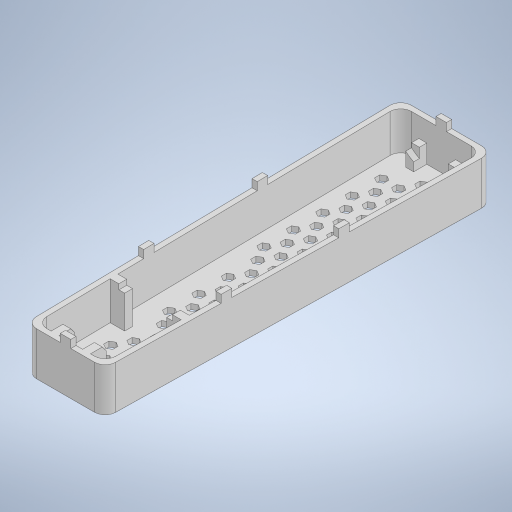
# Autodesk Inventor part: ContainerBottom
Saved by Autodesk Inventor 2023 (Build 270158000, 158)
## iProperties
Created: 2022-11-08
Part Number: ContainerBottom
Material: Generic
Document SubType Name: Modeling
Designer: The-M-Factor
Density: 1 g/cm^3
Appearance: Default
Author: The-M-Factor
Autodesk Inventor part; units mm, degrees
ref_plane "YZ Plane" through (0, 0, 0) normal (1, 0, 0) x (0, 1, 0)
ref_plane "XZ Plane" through (0, 0, 0) normal (0, 1, 0) x (-1, 0, 0)
sketch "Sketch1" plane through (0, 0, 0) normal (0, 1, 0) x (-1, 0, 0)
  line L0 (0, 0) -> (35, 0)
  line L1 (31.0843, 145) -> (2.5, 145)
  line L2 (2.5, 145) -> (32.5, 145)
  line L3 (32.5, 145) -> (35, 0)
  line L4 (0, 0) -> (2.5, 145)
  line L5 (32.9652, 2) -> (2.0348, 2)
  line L6 (2.0348, 2) -> (4.4658, 143)
  line L7 (4.4658, 143) -> (30.5342, 143)
  line L8 (30.5342, 143) -> (32.9652, 2)
  line L9 (26, 6.9925) -> (23, 6.9925)
  line L10 (26, 6.9925) -> (26, 2)
  line L11 (23, 6.9925) -> (23, 2)
  line L12 (17.5, 2) -> (17.5, 5.1674)
  line L13 (9, 6.9925) -> (12, 6.9925)
  line L14 (9, 6.9925) -> (9, 2)
  line L15 (12, 6.9925) -> (12, 2)
  line L16 (25, 137.0075) -> (22, 137.0075)
  line L17 (22, 137.0075) -> (22, 143)
  line L18 (25, 137.0075) -> (25, 143)
  line L19 (17.5, 143) -> (17.5, 140.473)
  line L20 (10, 137.0075) -> (13, 137.0075)
  line L21 (13, 137.0075) -> (13, 143)
  line L22 (10, 137.0075) -> (10, 143)
  line L23 (25.5, 114.5) -> (25.5, 111.5)
  line L24 (25.5, 111.5) -> (31.0773, 111.5)
  line L25 (25.5, 114.5) -> (31.0256, 114.5)
  line L26 (9.5, 114.5) -> (9.5, 111.5)
  line L27 (9.5, 111.5) -> (3.9227, 111.5)
  line L28 (9.5, 114.5) -> (3.9744, 114.5)
  point P0 (24.5, 6.9925)
  point P1 (23.5, 137.0075)
  point P2 (25.5, 113)
  point P3 (3.9744, 114.5)
  point P4 (3.9227, 111.5)
  point P5 (9, 2)
  point P6 (12, 2)
  dimension "d0" = 35
  dimension "d1" = 30
  dimension "d2" = 145
  dimension "d3" = 2.5
  dimension "d4" = 2
  dimension "d5" = 7
  dimension "d6" = 4.9925
  dimension "d8" = 3.1674
  dimension "d9" = 90
  dimension "d10" = 3
  dimension "d11" = 3
  dimension "d12" = 6
  dimension "d13" = 5.9925
  dimension "d14" = 3
  dimension "d15" = 30
  dimension "d16" = 8
  constraints: 58 end point, 12 symmetric about line, 7 point on line, 5 horizontal, 5 midpoint, 4 perpendicular, 2 vertical, 1 parallel, 3 other
  measures "d0" distance of L0.start L0.end
  measures "d1" distance of L1.end L2.end
  measures "d2" distance between parallel lines of L0 L1
  measures "d3" horizontal distance of L0.start L1.end
  measures "d4" distance between parallel lines of L3 L8
  measures "d5" horizontal distance of L12.start point (24.5, 6.992)
  measures "d6" vertical distance of L12.start point (24.5, 6.992)
  measures "d8" distance of L12.start L12.end
  measures "d9" angle of L5 L12
  measures "d10" distance of L16.start L16.end
  measures "d11" distance of L9.start L9.end
  measures "d12" horizontal distance of L19.start point (23.5, 137.008)
  measures "d13" vertical distance of L19.start point (23.5, 137.008)
  measures "d14" distance of L23.start L23.end
  measures "d15" vertical distance of L19.start point (25.5, 113)
  measures "d16" horizontal distance of L19.start point (25.5, 113)
extrude "Extrusion1" add sketch "Sketch1" along normal blind 2 contours L5 L10 L9 L11 L15 L13 L14 L6 L27 L26 L28 L7 L22 L20 L21 L17 L16 L18 L8 L25 L23 L24
extrude "Extrusion2" add sketch "Sketch1" along normal blind 16.5
extrude "Extrusion3" add sketch "Sketch1" along normal blind 16.5 contours L24 L23 L25 L8
extrude "Extrusion4" add sketch "Sketch1" along normal blind 16.5 contours L6 L28 L26 L27
extrude "Extrusion5" add sketch "Sketch1" along normal blind 16.5 contours L18 L16 L17 L7
extrude "Extrusion6" add sketch "Sketch1" along normal blind 16.5 contours L21 L20 L22 L7
extrude "Extrusion7" add sketch "Sketch1" along normal blind 9 contours L5 L11 L9 L10
extrude "Extrusion8" add sketch "Sketch1" along normal blind 9 contours L5 L14 L13 L15
sketch "Sketch2" plane through (0, 16.5, 0) normal (0, 1, 0) x (1, 0, 0)
  line L0 (-31.0256, -114.5) -> (-25.5, -114.5) projected
  line L1 (-27.7, -114.5) -> (-27.7, -111.5)
  line L2 (-25.5, -111.5) -> (-31.0773, -111.5) projected
  line L3 (-25.5, -114.5) -> (-25.5, -111.5) projected
  line L4 (-9.5, -114.5) -> (-3.9744, -114.5) projected
  line L5 (-7.3, -114.5) -> (-7.3, -111.5)
  line L6 (-3.9227, -111.5) -> (-9.5, -111.5) projected
  line L7 (-9.5, -111.5) -> (-9.5, -114.5) projected
  point P0 (0, 0)
  dimension "d33" = 2.2
  dimension "d34" = 2.2
  constraints: 4 end point, 4 point on line, 2 vertical
  measures "d33" distance between parallel lines of L3 L1
  measures "d34" distance between parallel lines of L7 L5
extrude "Extrusion9" cut sketch "Sketch2" against normal blind 2 contours L1 L2 L3 L0
extrude "Extrusion10" cut sketch "Sketch2" against normal blind 2 contours L7 L6 L5 L4
chamfer "Chamfer1" distance 1.5 distance2 2 1 edges at (-11.5, 16.5, 137.0075) measured on face at (-2.1409, 16.5, 85.5)
chamfer "Chamfer2" distance 1.5 distance2 2 1 edges at (-23.5, 16.5, 137.0075) measured on face at (-2.1409, 16.5, 85.5)
ref_plane "Work Plane1" through (0, 0, 6.9925) normal (0, 0, 1) x (1, 0, 0)
sketch "Sketch3" plane through (0, 0, 6.9925) normal (0, 0, 1) x (1, 0, 0)
  line L0 (-12, 2) -> (-12, 9) projected
  line L1 (-23, 2) -> (-12, 2)
  line L2 (-17.5, 2) -> (-17.5, 16.5)
  circle A0 centre (-17.5, 16.5) radius 12.5
  point P0 (0, 0)
  dimension "d46" = 14.5
  dimension "d47" = 25
  constraints: 4 end point, 1 centre point, 1 coincident, 1 horizontal, 1 midpoint, 1 vertical
  measures "d46" distance of L2.start L2.end
  measures "d47" diameter of A0
extrude "Extrusion11" cut sketch "Sketch3" against normal blind 2.2 contours A0
sketch "Sketch5" plane through (0, 2, 0) normal (0, 1, 0) x (1, 0, 0)
  line L0 (-17, -131) -> (-15.2679, -132)
  line L1 (-15.2679, -132) -> (-15.2679, -134)
  line L2 (-15.2679, -134) -> (-17, -135)
  line L3 (-17, -135) -> (-18.7321, -134)
  line L4 (-18.7321, -134) -> (-18.7321, -132)
  line L5 (-18.7321, -132) -> (-17, -131)
  line L6 (-22, -137.0075) -> (-22, -143) projected
  line L7 (-22, -143) -> (-13, -143) projected
  line L8 (-22.1856, -132.2619) -> (-19.9814, -130.9893)
  line L9 (-14.5757, -130.6676) -> (-12.1577, -132.0636)
  line L10 (-18.7321, -133) -> (-19.3956, -133)
  line L11 (-25.5, -111.5) -> (-25.5, -114.5) projected
  line L12 (-32.9652, -2) -> (-31.0773, -111.5) projected
  line L13 (-15.5, -128.4019) -> (-13.7679, -129.4019)
  line L14 (-13.7679, -129.4019) -> (-12.0359, -128.4019)
  line L15 (-12.0359, -128.4019) -> (-12.0359, -126.4019)
  line L16 (-12.0359, -126.4019) -> (-13.7679, -125.4019)
  line L17 (-13.7679, -125.4019) -> (-15.5, -126.4019)
  line L18 (-15.5, -126.4019) -> (-15.5, -128.4019)
  line L19 (-18.5, -128.4019) -> (-18.5, -126.4019)
  line L20 (-18.5, -126.4019) -> (-20.2321, -125.4019)
  line L21 (-20.2321, -125.4019) -> (-21.9641, -126.4019)
  line L22 (-21.9641, -126.4019) -> (-21.9641, -128.4019)
  line L23 (-21.9641, -128.4019) -> (-20.2321, -129.4019)
  line L24 (-20.2321, -129.4019) -> (-18.5, -128.4019)
  line L25 (-18.2258, -127.4019) -> (-16.8285, -127.4019)
  line L26 (-17, -123.8038) -> (-15.2679, -122.8038)
  line L27 (-15.2679, -122.8038) -> (-15.2679, -120.8038)
  line L28 (-15.2679, -120.8038) -> (-17, -119.8038)
  line L29 (-17, -119.8038) -> (-18.7321, -120.8038)
  line L30 (-18.7321, -120.8038) -> (-18.7321, -122.8038)
  line L31 (-18.7321, -122.8038) -> (-17, -123.8038)
  line L32 (-18.7321, -121.8038) -> (-20.5, -121.8038)
  line L33 (-17, -112.6077) -> (-15.2679, -111.6077)
  line L34 (-15.2679, -111.6077) -> (-15.2679, -109.6077)
  line L35 (-15.2679, -109.6077) -> (-17, -108.6077)
  line L36 (-17, -108.6077) -> (-18.7321, -109.6077)
  line L37 (-18.7321, -109.6077) -> (-18.7321, -111.6077)
  line L38 (-18.7321, -111.6077) -> (-17, -112.6077)
  line L39 (-22.1856, -111.3458) -> (-19.9814, -112.6184)
  line L40 (-14.5757, -112.9401) -> (-12.1577, -111.5441)
  line L41 (-18.7321, -110.6077) -> (-19.3956, -110.6077)
  line L42 (-13.7679, -118.2058) -> (-15.5, -117.2058)
  line L43 (-12.0359, -117.2058) -> (-13.7679, -118.2058)
  line L44 (-12.0359, -115.2058) -> (-12.0359, -117.2058)
  line L45 (-13.7679, -114.2058) -> (-12.0359, -115.2058)
  line L46 (-15.5, -115.2058) -> (-13.7679, -114.2058)
  line L47 (-15.5, -117.2058) -> (-15.5, -115.2058)
  line L48 (-21.9641, -115.2058) -> (-20.2321, -114.2058)
  line L49 (-21.9641, -117.2058) -> (-21.9641, -115.2058)
  line L50 (-20.2321, -118.2058) -> (-21.9641, -117.2058)
  line L51 (-18.5, -117.2058) -> (-20.2321, -118.2058)
  line L52 (-18.5, -115.2058) -> (-18.5, -117.2058)
  line L53 (-20.2321, -114.2058) -> (-18.5, -115.2058)
  line L54 (-18.2258, -116.2058) -> (-16.8285, -116.2058)
  line L55 (-18.7321, -98.4115) -> (-17, -97.4115)
  line L56 (-18.7321, -100.4115) -> (-18.7321, -98.4115)
  line L57 (-17, -101.4115) -> (-18.7321, -100.4115)
  line L58 (-15.2679, -100.4115) -> (-17, -101.4115)
  line L59 (-15.2679, -98.4115) -> (-15.2679, -100.4115)
  line L60 (-17, -97.4115) -> (-15.2679, -98.4115)
  line L61 (-18.7321, -99.4115) -> (-20.5, -99.4115)
  line L62 (-21.9641, -104.0096) -> (-21.9641, -106.0096)
  line L63 (-18.5, -104.0096) -> (-20.2321, -103.0096)
  line L64 (-20.2321, -103.0096) -> (-21.9641, -104.0096)
  line L65 (-21.9641, -106.0096) -> (-20.2321, -107.0096)
  line L66 (-18.5, -106.0096) -> (-18.5, -104.0096)
  line L67 (-20.2321, -107.0096) -> (-18.5, -106.0096)
  line L68 (-18.2258, -105.0096) -> (-16.8285, -105.0096)
  line L69 (-13.7679, -107.0096) -> (-12.0359, -106.0096)
  line L70 (-13.7679, -103.0096) -> (-15.5, -104.0096)
  line L71 (-12.0359, -106.0096) -> (-12.0359, -104.0096)
  line L72 (-12.0359, -104.0096) -> (-13.7679, -103.0096)
  line L73 (-15.5, -106.0096) -> (-13.7679, -107.0096)
  line L74 (-15.5, -104.0096) -> (-15.5, -106.0096)
  line L75 (-22.1856, -109.8696) -> (-19.9814, -108.597)
  line L76 (-14.5757, -108.2753) -> (-12.1577, -109.6713)
  line L77 (-18.7321, -76.0192) -> (-17, -75.0192)
  line L78 (-18.7321, -78.0192) -> (-18.7321, -76.0192)
  line L79 (-17, -79.0192) -> (-18.7321, -78.0192)
  line L80 (-15.2679, -78.0192) -> (-17, -79.0192)
  line L81 (-15.2679, -76.0192) -> (-15.2679, -78.0192)
  line L82 (-17, -75.0192) -> (-15.2679, -76.0192)
  line L83 (-18.7321, -77.0192) -> (-20.5, -77.0192)
  line L84 (-21.9641, -81.6173) -> (-21.9641, -83.6173)
  line L85 (-18.5, -81.6173) -> (-20.2321, -80.6173)
  line L86 (-20.2321, -80.6173) -> (-21.9641, -81.6173)
  line L87 (-21.9641, -83.6173) -> (-20.2321, -84.6173)
  line L88 (-18.5, -83.6173) -> (-18.5, -81.6173)
  line L89 (-20.2321, -84.6173) -> (-18.5, -83.6173)
  line L90 (-18.2258, -82.6173) -> (-16.8285, -82.6173)
  line L91 (-13.7679, -84.6173) -> (-12.0359, -83.6173)
  line L92 (-13.7679, -80.6173) -> (-15.5, -81.6173)
  line L93 (-12.0359, -83.6173) -> (-12.0359, -81.6173)
  line L94 (-12.0359, -81.6173) -> (-13.7679, -80.6173)
  line L95 (-15.5, -83.6173) -> (-13.7679, -84.6173)
  line L96 (-15.5, -81.6173) -> (-15.5, -83.6173)
  line L97 (-22.1856, -87.4773) -> (-19.9814, -86.2047)
  line L98 (-14.5757, -85.883) -> (-12.1577, -87.279)
  line L99 (-17, -86.2154) -> (-15.2679, -87.2154)
  line L100 (-18.7321, -87.2154) -> (-17, -86.2154)
  line L101 (-18.7321, -89.2154) -> (-18.7321, -87.2154)
  line L102 (-17, -90.2154) -> (-18.7321, -89.2154)
  line L103 (-15.2679, -89.2154) -> (-17, -90.2154)
  line L104 (-15.2679, -87.2154) -> (-15.2679, -89.2154)
  line L105 (-18.7321, -88.2154) -> (-19.3956, -88.2154)
  line L106 (-20.2321, -95.8135) -> (-21.9641, -94.8135)
  line L107 (-18.5, -94.8135) -> (-20.2321, -95.8135)
  line L108 (-14.5757, -90.5478) -> (-12.1577, -89.1518)
  line L109 (-15.5, -92.8135) -> (-13.7679, -91.8135)
  line L110 (-13.7679, -95.8135) -> (-15.5, -94.8135)
  line L111 (-12.0359, -94.8135) -> (-13.7679, -95.8135)
  line L112 (-12.0359, -92.8135) -> (-12.0359, -94.8135)
  line L113 (-13.7679, -91.8135) -> (-12.0359, -92.8135)
  line L114 (-15.5, -94.8135) -> (-15.5, -92.8135)
  line L115 (-18.2258, -93.8135) -> (-16.8285, -93.8135)
  line L116 (-21.9641, -94.8135) -> (-21.9641, -92.8135)
  line L117 (-18.5, -92.8135) -> (-18.5, -94.8135)
  line L118 (-21.9641, -92.8135) -> (-20.2321, -91.8135)
  line L119 (-20.2321, -91.8135) -> (-18.5, -92.8135)
  line L120 (-22.1856, -88.9535) -> (-19.9814, -90.2261)
  line L121 (-18.7321, -31.2346) -> (-17, -30.2346)
  line L122 (-18.7321, -33.2346) -> (-18.7321, -31.2346)
  line L123 (-17, -34.2346) -> (-18.7321, -33.2346)
  line L124 (-15.2679, -33.2346) -> (-17, -34.2346)
  line L125 (-15.2679, -31.2346) -> (-15.2679, -33.2346)
  line L126 (-17, -30.2346) -> (-15.2679, -31.2346)
  line L127 (-18.7321, -32.2346) -> (-20.5, -32.2346)
  line L128 (-21.9641, -36.8327) -> (-21.9641, -38.8327)
  line L129 (-18.5, -36.8327) -> (-20.2321, -35.8327)
  line L130 (-20.2321, -35.8327) -> (-21.9641, -36.8327)
  line L131 (-21.9641, -38.8327) -> (-20.2321, -39.8327)
  line L132 (-18.5, -38.8327) -> (-18.5, -36.8327)
  line L133 (-20.2321, -39.8327) -> (-18.5, -38.8327)
  line L134 (-18.2258, -37.8327) -> (-16.8285, -37.8327)
  line L135 (-13.7679, -39.8327) -> (-12.0359, -38.8327)
  line L136 (-13.7679, -35.8327) -> (-15.5, -36.8327)
  line L137 (-12.0359, -38.8327) -> (-12.0359, -36.8327)
  line L138 (-12.0359, -36.8327) -> (-13.7679, -35.8327)
  line L139 (-15.5, -38.8327) -> (-13.7679, -39.8327)
  line L140 (-15.5, -36.8327) -> (-15.5, -38.8327)
  line L141 (-22.1856, -42.6927) -> (-19.9814, -41.4201)
  line L142 (-14.5757, -41.0984) -> (-12.1577, -42.4944)
  line L143 (-17, -41.4308) -> (-15.2679, -42.4308)
  line L144 (-18.7321, -42.4308) -> (-17, -41.4308)
  line L145 (-18.7321, -44.4308) -> (-18.7321, -42.4308)
  line L146 (-17, -45.4308) -> (-18.7321, -44.4308)
  line L147 (-15.2679, -44.4308) -> (-17, -45.4308)
  line L148 (-15.2679, -42.4308) -> (-15.2679, -44.4308)
  line L149 (-18.7321, -43.4308) -> (-19.3956, -43.4308)
  line L150 (-18.7321, -55.6269) -> (-17, -56.6269)
  line L151 (-17, -56.6269) -> (-15.2679, -55.6269)
  line L152 (-18.7321, -54.6269) -> (-20.5, -54.6269)
  line L153 (-18.7321, -53.6269) -> (-18.7321, -55.6269)
  line L154 (-15.2679, -55.6269) -> (-15.2679, -53.6269)
  line L155 (-15.2679, -53.6269) -> (-17, -52.6269)
  line L156 (-17, -52.6269) -> (-18.7321, -53.6269)
  line L157 (-20.2321, -51.0289) -> (-21.9641, -50.0289)
  line L158 (-18.5, -50.0289) -> (-20.2321, -51.0289)
  line L159 (-14.5757, -45.7632) -> (-12.1577, -44.3671)
  line L160 (-15.5, -48.0289) -> (-13.7679, -47.0289)
  line L161 (-13.7679, -51.0289) -> (-15.5, -50.0289)
  line L162 (-12.0359, -50.0289) -> (-13.7679, -51.0289)
  line L163 (-12.0359, -48.0289) -> (-12.0359, -50.0289)
  line L164 (-13.7679, -47.0289) -> (-12.0359, -48.0289)
  line L165 (-15.5, -50.0289) -> (-15.5, -48.0289)
  line L166 (-18.2258, -49.0289) -> (-16.8285, -49.0289)
  line L167 (-21.9641, -50.0289) -> (-21.9641, -48.0289)
  line L168 (-18.5, -48.0289) -> (-18.5, -50.0289)
  line L169 (-21.9641, -48.0289) -> (-20.2321, -47.0289)
  line L170 (-20.2321, -47.0289) -> (-18.5, -48.0289)
  line L171 (-22.1856, -44.1689) -> (-19.9814, -45.4415)
  line L172 (-20.2321, -69.4212) -> (-18.5, -70.4212)
  line L173 (-21.9641, -70.4212) -> (-20.2321, -69.4212)
  line L174 (-18.5, -72.4212) -> (-20.2321, -73.4212)
  line L175 (-21.9641, -72.4212) -> (-21.9641, -70.4212)
  line L176 (-20.2321, -73.4212) -> (-21.9641, -72.4212)
  line L177 (-18.5, -61.225) -> (-18.5, -59.225)
  line L178 (-22.1856, -65.085) -> (-19.9814, -63.8124)
  line L179 (-18.2258, -71.4212) -> (-16.8285, -71.4212)
  line L180 (-18.5, -70.4212) -> (-18.5, -72.4212)
  line L181 (-13.7679, -73.4212) -> (-15.5, -72.4212)
  line L182 (-12.0359, -72.4212) -> (-13.7679, -73.4212)
  line L183 (-15.5, -72.4212) -> (-15.5, -70.4212)
  line L184 (-12.0359, -70.4212) -> (-12.0359, -72.4212)
  line L185 (-15.5, -70.4212) -> (-13.7679, -69.4212)
  line L186 (-13.7679, -69.4212) -> (-12.0359, -70.4212)
  line L187 (-22.1856, -66.5612) -> (-19.9814, -67.8338)
  line L188 (-18.7321, -66.8231) -> (-17, -67.8231)
  line L189 (-14.5757, -68.1555) -> (-12.1577, -66.7594)
  line L190 (-17, -67.8231) -> (-15.2679, -66.8231)
  line L191 (-18.7321, -64.8231) -> (-18.7321, -66.8231)
  line L192 (-15.2679, -66.8231) -> (-15.2679, -64.8231)
  line L193 (-17, -63.8231) -> (-18.7321, -64.8231)
  line L194 (-15.2679, -64.8231) -> (-17, -63.8231)
  line L195 (-18.7321, -65.8231) -> (-19.3956, -65.8231)
  line L196 (-18.5, -59.225) -> (-20.2321, -58.225)
  line L197 (-20.2321, -58.225) -> (-21.9641, -59.225)
  line L198 (-21.9641, -61.225) -> (-20.2321, -62.225)
  line L199 (-21.9641, -59.225) -> (-21.9641, -61.225)
  line L200 (-20.2321, -62.225) -> (-18.5, -61.225)
  line L201 (-14.5757, -63.4907) -> (-12.1577, -64.8867)
  line L202 (-18.2258, -60.225) -> (-16.8285, -60.225)
  line L203 (-15.5, -61.225) -> (-13.7679, -62.225)
  line L204 (-13.7679, -62.225) -> (-12.0359, -61.225)
  line L205 (-15.5, -59.225) -> (-15.5, -61.225)
  line L206 (-12.0359, -61.225) -> (-12.0359, -59.225)
  line L207 (-12.0359, -59.225) -> (-13.7679, -58.225)
  line L208 (-13.7679, -58.225) -> (-15.5, -59.225)
  line L209 (-18.5, -27.6366) -> (-20.2321, -28.6366)
  line L210 (-20.2321, -28.6366) -> (-21.9641, -27.6366)
  line L211 (-21.9641, -27.6366) -> (-21.9641, -25.6366)
  line L212 (-20.2321, -24.6366) -> (-18.5, -25.6366)
  line L213 (-21.9641, -25.6366) -> (-20.2321, -24.6366)
  line L214 (-22.1856, -21.7766) -> (-19.9814, -23.0492)
  line L215 (-18.7321, -22.0385) -> (-17, -23.0385)
  line L216 (-18.7321, -21.0385) -> (-19.3956, -21.0385)
  line L217 (-14.5757, -23.3709) -> (-12.1577, -21.9748)
  line L218 (-18.7321, -20.0385) -> (-18.7321, -22.0385)
  line L219 (-17, -23.0385) -> (-15.2679, -22.0385)
  line L220 (-15.2679, -22.0385) -> (-15.2679, -20.0385)
  line L221 (-17, -19.0385) -> (-18.7321, -20.0385)
  line L222 (-15.2679, -20.0385) -> (-17, -19.0385)
  line L223 (-22.1856, -20.3004) -> (-19.9814, -19.0278)
  line L224 (-18.2258, -15.4404) -> (-16.8285, -15.4404)
  line L225 (-20.2321, -17.4404) -> (-18.5, -16.4404)
  line L226 (-21.9641, -16.4404) -> (-20.2321, -17.4404)
  line L227 (-18.5, -16.4404) -> (-18.5, -14.4404)
  line L228 (-18.5, -14.4404) -> (-20.2321, -13.4404)
  line L229 (-21.9641, -14.4404) -> (-21.9641, -16.4404)
  line L230 (-20.2321, -13.4404) -> (-21.9641, -14.4404)
  line L231 (-18.5, -25.6366) -> (-18.5, -27.6366)
  line L232 (-18.2258, -26.6366) -> (-16.8285, -26.6366)
  line L233 (-15.5, -25.6366) -> (-13.7679, -24.6366)
  line L234 (-15.5, -27.6366) -> (-15.5, -25.6366)
  line L235 (-13.7679, -28.6366) -> (-15.5, -27.6366)
  line L236 (-12.0359, -25.6366) -> (-12.0359, -27.6366)
  line L237 (-12.0359, -27.6366) -> (-13.7679, -28.6366)
  line L238 (-13.7679, -24.6366) -> (-12.0359, -25.6366)
  line L239 (-18.7321, -8.8423) -> (-17, -7.8423)
  line L240 (-17, -7.8423) -> (-15.2679, -8.8423)
  line L241 (-18.7321, -9.8423) -> (-20.5, -9.8423)
  line L242 (-18.7321, -10.8423) -> (-18.7321, -8.8423)
  line L243 (-15.2679, -8.8423) -> (-15.2679, -10.8423)
  line L244 (-15.2679, -10.8423) -> (-17, -11.8423)
  line L245 (-17, -11.8423) -> (-18.7321, -10.8423)
  line L246 (-14.5757, -18.7061) -> (-12.1577, -20.1021)
  line L247 (-15.5, -16.4404) -> (-13.7679, -17.4404)
  line L248 (-15.5, -14.4404) -> (-15.5, -16.4404)
  line L249 (-13.7679, -17.4404) -> (-12.0359, -16.4404)
  line L250 (-12.0359, -16.4404) -> (-12.0359, -14.4404)
  line L251 (-12.0359, -14.4404) -> (-13.7679, -13.4404)
  line L252 (-13.7679, -13.4404) -> (-15.5, -14.4404)
  line L253 (-25.5, -114.5) -> (-31.0256, -114.5) projected
  point P0 (0, 0)
  point P1 (-17, -133)
  point P2 (-21.0835, -131.6256)
  point P3 (-19.0638, -133)
  dimension "d55" = 2
  dimension "d59" = 1.5
  dimension "d60" = 1.5
  dimension "d63" = 2.0638
  dimension "d170" = 3.5981
  dimension "d184" = 8.5
  dimension "d185" = 18.5
  dimension "d186" = 90
  constraints: 498 end point, 278 symmetric about line, 4 midpoint, 3 horizontal, 2 parallel, 13 other
  measures "d55" distance of L0.end L1.end
  measures "d59" distance from line of L5 point (-21.084, -131.626)
  measures "d60" distance between parallel lines of L0 L9
  measures "d63" horizontal distance of L0.start point (-19.064, -133)
  measures "d170" vertical distance of L0.start L25.start
  measures "d184" distance from line of L11 point (-17, -133)
  measures "d185" distance from line of L253 point (-17, -133)
  measures "d186" angle of L253 L4
fillet "Fillet1" radius 4 2 edges at (-35, 8.25, 0) (0, 8.25, 0)
fillet "Fillet2" radius 4 1 edges at (-32.9652, 9.25, 2)
fillet "Fillet3" radius 4 1 edges at (-2.0348, 9.25, 2)
fillet "Fillet4" radius 4 2 edges at (-32.5, 8.25, 145) (-2.5, 8.25, 145)
fillet "Fillet5" radius 4 1 edges at (-30.5342, 9.25, 143)
fillet "Fillet6" radius 4 1 edges at (-4.4658, 9.25, 143)
extrude "CenterHoles" cut sketch "Sketch5" against normal blind 2
sketch "Sketch8" plane through (0, 2, 0) normal (0, 1, 0) x (1, 0, 0)
  line L0 (-24.9641, -14.4404) -> (-24.9641, -16.4404)
  line L1 (-24.9641, -16.4404) -> (-26.6962, -17.4404)
  line L2 (-26.6962, -17.4404) -> (-28.4282, -16.4404)
  line L3 (-28.4282, -16.4404) -> (-28.4282, -14.4404)
  line L4 (-28.4282, -14.4404) -> (-26.6962, -13.4404)
  line L5 (-26.6962, -13.4404) -> (-24.9641, -14.4404)
  line L6 (-26, -6.9925) -> (-26, -4.7925) projected
  line L7 (-21.9641, -16.4404) -> (-21.9641, -14.4404) projected
  line L8 (-26.8244, -19.2465) -> (-24.0082, -17.6206)
  line L9 (-21.7321, -20.0385) -> (-23.4641, -19.0385)
  line L10 (-23.4641, -19.0385) -> (-25.1962, -20.0385)
  line L11 (-25.1962, -20.0385) -> (-25.1962, -22.0385)
  line L12 (-25.1962, -22.0385) -> (-23.4641, -23.0385)
  line L13 (-23.4641, -23.0385) -> (-21.7321, -22.0385)
  line L14 (-21.7321, -22.0385) -> (-21.7321, -20.0385)
  line L15 (-25.1962, -21.0385) -> (-26.7131, -21.0385)
  line L16 (-24.9641, -27.6366) -> (-24.9641, -25.6366)
  line L17 (-24.9641, -25.6366) -> (-26.6962, -24.6366)
  line L18 (-26.6962, -24.6366) -> (-28.4282, -25.6366)
  line L19 (-28.4282, -25.6366) -> (-28.4282, -27.6366)
  line L20 (-28.4282, -27.6366) -> (-26.6962, -28.6366)
  line L21 (-26.6962, -28.6366) -> (-24.9641, -27.6366)
  line L22 (-26.8244, -22.8304) -> (-24.0082, -24.4564)
  line L23 (-24.9641, -26.6366) -> (-24.1308, -26.6366)
  line L24 (-24.9641, -38.8327) -> (-24.9641, -36.8327)
  line L25 (-24.9641, -36.8327) -> (-26.6962, -35.8327)
  line L26 (-26.6962, -35.8327) -> (-28.4282, -36.8327)
  line L27 (-28.4282, -36.8327) -> (-28.4282, -38.8327)
  line L28 (-28.4282, -38.8327) -> (-26.6962, -39.8327)
  line L29 (-26.6962, -39.8327) -> (-24.9641, -38.8327)
  line L30 (-26.8244, -34.0266) -> (-24.0082, -35.6525)
  line L31 (-21.7321, -31.2346) -> (-21.7321, -33.2346)
  line L32 (-21.7321, -33.2346) -> (-23.4641, -34.2346)
  line L33 (-23.4641, -34.2346) -> (-25.1962, -33.2346)
  line L34 (-25.1962, -33.2346) -> (-25.1962, -31.2346)
  line L35 (-25.1962, -31.2346) -> (-23.4641, -30.2346)
  line L36 (-23.4641, -30.2346) -> (-21.7321, -31.2346)
  line L37 (-25.1962, -32.2346) -> (-26.7131, -32.2346)
  line L38 (-26.8244, -30.4427) -> (-24.0082, -28.8167)
  line L39 (-24.9641, -37.8327) -> (-24.1308, -37.8327)
  line L40 (-21.7321, -53.6269) -> (-21.7321, -55.6269)
  line L41 (-21.7321, -55.6269) -> (-23.4641, -56.6269)
  line L42 (-23.4641, -56.6269) -> (-25.1962, -55.6269)
  line L43 (-25.1962, -55.6269) -> (-25.1962, -53.6269)
  line L44 (-25.1962, -53.6269) -> (-23.4641, -52.6269)
  line L45 (-23.4641, -52.6269) -> (-21.7321, -53.6269)
  line L46 (-25.1962, -54.6269) -> (-26.7131, -54.6269)
  line L47 (-28.4282, -50.0289) -> (-28.4282, -48.0289)
  line L48 (-28.4282, -48.0289) -> (-26.6962, -47.0289)
  line L49 (-26.6962, -47.0289) -> (-24.9641, -48.0289)
  line L50 (-24.9641, -48.0289) -> (-24.9641, -50.0289)
  line L51 (-24.9641, -50.0289) -> (-26.6962, -51.0289)
  line L52 (-26.6962, -51.0289) -> (-28.4282, -50.0289)
  line L53 (-26.8244, -52.835) -> (-24.0082, -51.209)
  line L54 (-24.9641, -49.0289) -> (-24.1308, -49.0289)
  line L55 (-26.8244, -41.6388) -> (-24.0082, -40.0129)
  line L56 (-25.1962, -43.4308) -> (-26.7131, -43.4308)
  line L57 (-26.8244, -45.2228) -> (-24.0082, -46.8487)
  line L58 (-25.1962, -44.4308) -> (-23.4641, -45.4308)
  line L59 (-25.1962, -42.4308) -> (-25.1962, -44.4308)
  line L60 (-23.4641, -41.4308) -> (-25.1962, -42.4308)
  line L61 (-21.7321, -42.4308) -> (-23.4641, -41.4308)
  line L62 (-21.7321, -44.4308) -> (-21.7321, -42.4308)
  line L63 (-23.4641, -45.4308) -> (-21.7321, -44.4308)
  line L64 (-26.8244, -56.4189) -> (-24.0082, -58.0448)
  line L65 (-24.9641, -60.225) -> (-24.1308, -60.225)
  line L66 (-28.4282, -61.225) -> (-26.6962, -62.225)
  line L67 (-26.6962, -62.225) -> (-24.9641, -61.225)
  line L68 (-24.9641, -61.225) -> (-24.9641, -59.225)
  line L69 (-26.6962, -58.225) -> (-28.4282, -59.225)
  line L70 (-24.9641, -59.225) -> (-26.6962, -58.225)
  line L71 (-28.4282, -59.225) -> (-28.4282, -61.225)
  line L72 (-25.1962, -64.8231) -> (-23.4641, -63.8231)
  line L73 (-23.4641, -63.8231) -> (-21.7321, -64.8231)
  line L74 (-25.1962, -65.8231) -> (-26.7131, -65.8231)
  line L75 (-25.1962, -66.8231) -> (-25.1962, -64.8231)
  line L76 (-21.7321, -64.8231) -> (-21.7321, -66.8231)
  line L77 (-21.7321, -66.8231) -> (-23.4641, -67.8231)
  line L78 (-23.4641, -67.8231) -> (-25.1962, -66.8231)
  line L79 (-23.4641, -75.0192) -> (-25.1962, -76.0192)
  line L80 (-21.7321, -76.0192) -> (-23.4641, -75.0192)
  line L81 (-25.1962, -77.0192) -> (-26.7131, -77.0192)
  line L82 (-21.7321, -78.0192) -> (-21.7321, -76.0192)
  line L83 (-23.4641, -79.0192) -> (-21.7321, -78.0192)
  line L84 (-25.1962, -76.0192) -> (-25.1962, -78.0192)
  line L85 (-25.1962, -78.0192) -> (-23.4641, -79.0192)
  line L86 (-25.1962, -87.2154) -> (-23.4641, -86.2154)
  line L87 (-23.4641, -86.2154) -> (-21.7321, -87.2154)
  line L88 (-25.1962, -88.2154) -> (-26.7131, -88.2154)
  line L89 (-25.1962, -89.2154) -> (-25.1962, -87.2154)
  line L90 (-21.7321, -87.2154) -> (-21.7321, -89.2154)
  line L91 (-21.7321, -89.2154) -> (-23.4641, -90.2154)
  line L92 (-23.4641, -90.2154) -> (-25.1962, -89.2154)
  line L93 (-23.4641, -101.4115) -> (-25.1962, -100.4115)
  line L94 (-25.1962, -98.4115) -> (-23.4641, -97.4115)
  line L95 (-25.1962, -99.4115) -> (-26.7131, -99.4115)
  line L96 (-23.4641, -97.4115) -> (-21.7321, -98.4115)
  line L97 (-25.1962, -100.4115) -> (-25.1962, -98.4115)
  line L98 (-21.7321, -100.4115) -> (-23.4641, -101.4115)
  line L99 (-21.7321, -98.4115) -> (-21.7321, -100.4115)
  line L100 (-17, -75.0192) -> (-17, -73.4581)
  line L101 (-15.2679, -76.0192) -> (-15.2679, -78.0192) projected
  line L102 (-23.4641, -123.8038) -> (-25.1962, -122.8038)
  line L103 (-25.1962, -120.8038) -> (-23.4641, -119.8038)
  line L104 (-25.1962, -121.8038) -> (-26.7131, -121.8038)
  line L105 (-23.4641, -119.8038) -> (-21.7321, -120.8038)
  line L106 (-25.1962, -122.8038) -> (-25.1962, -120.8038)
  line L107 (-21.7321, -122.8038) -> (-23.4641, -123.8038)
  line L108 (-21.7321, -120.8038) -> (-21.7321, -122.8038)
  line L109 (-9.0359, -14.4404) -> (-9.0359, -16.4404)
  line L110 (-9.0359, -16.4404) -> (-7.3038, -17.4404)
  line L111 (-7.3038, -17.4404) -> (-5.5718, -16.4404)
  line L112 (-5.5718, -16.4404) -> (-5.5718, -14.4404)
  line L113 (-5.5718, -14.4404) -> (-7.3038, -13.4404)
  line L114 (-7.3038, -13.4404) -> (-9.0359, -14.4404)
  line L115 (-7.1756, -19.2465) -> (-9.9918, -17.6206)
  line L116 (-12.2679, -22.0385) -> (-12.2679, -20.0385)
  line L117 (-12.2679, -20.0385) -> (-10.5359, -19.0385)
  line L118 (-10.5359, -19.0385) -> (-8.8038, -20.0385)
  line L119 (-8.8038, -20.0385) -> (-8.8038, -22.0385)
  line L120 (-8.8038, -22.0385) -> (-10.5359, -23.0385)
  line L121 (-10.5359, -23.0385) -> (-12.2679, -22.0385)
  line L122 (-8.8038, -21.0385) -> (-7.2869, -21.0385)
  line L123 (-5.5718, -25.6366) -> (-5.5718, -27.6366)
  line L124 (-5.5718, -27.6366) -> (-7.3038, -28.6366)
  line L125 (-7.3038, -28.6366) -> (-9.0359, -27.6366)
  line L126 (-9.0359, -27.6366) -> (-9.0359, -25.6366)
  line L127 (-9.0359, -25.6366) -> (-7.3038, -24.6366)
  line L128 (-7.3038, -24.6366) -> (-5.5718, -25.6366)
  line L129 (-7.1756, -22.8304) -> (-9.9918, -24.4564)
  line L130 (-9.0359, -26.6366) -> (-9.8692, -26.6366)
  line L131 (-9.0359, -38.8327) -> (-9.0359, -36.8327)
  line L132 (-7.3038, -39.8327) -> (-9.0359, -38.8327)
  line L133 (-5.5718, -38.8327) -> (-7.3038, -39.8327)
  line L134 (-5.5718, -36.8327) -> (-5.5718, -38.8327)
  line L135 (-7.3038, -35.8327) -> (-5.5718, -36.8327)
  line L136 (-9.0359, -36.8327) -> (-7.3038, -35.8327)
  line L137 (-7.1756, -34.0266) -> (-9.9918, -35.6525)
  line L138 (-8.8038, -32.2346) -> (-7.2869, -32.2346)
  line L139 (-7.1756, -30.4427) -> (-9.9918, -28.8167)
  line L140 (-8.8038, -31.2346) -> (-10.5359, -30.2346)
  line L141 (-8.8038, -33.2346) -> (-8.8038, -31.2346)
  line L142 (-10.5359, -34.2346) -> (-8.8038, -33.2346)
  line L143 (-12.2679, -33.2346) -> (-10.5359, -34.2346)
  line L144 (-12.2679, -31.2346) -> (-12.2679, -33.2346)
  line L145 (-10.5359, -30.2346) -> (-12.2679, -31.2346)
  line L146 (-9.0359, -37.8327) -> (-9.8692, -37.8327)
  line L147 (-10.5359, -56.6269) -> (-8.8038, -55.6269)
  line L148 (-12.2679, -55.6269) -> (-10.5359, -56.6269)
  line L149 (-8.8038, -54.6269) -> (-7.2869, -54.6269)
  line L150 (-12.2679, -53.6269) -> (-12.2679, -55.6269)
  line L151 (-10.5359, -52.6269) -> (-12.2679, -53.6269)
  line L152 (-8.8038, -55.6269) -> (-8.8038, -53.6269)
  line L153 (-8.8038, -53.6269) -> (-10.5359, -52.6269)
  line L154 (-7.1756, -52.835) -> (-9.9918, -51.209)
  line L155 (-9.0359, -49.0289) -> (-9.8692, -49.0289)
  line L156 (-5.5718, -48.0289) -> (-7.3038, -47.0289)
  line L157 (-7.3038, -47.0289) -> (-9.0359, -48.0289)
  line L158 (-9.0359, -48.0289) -> (-9.0359, -50.0289)
  line L159 (-7.3038, -51.0289) -> (-5.5718, -50.0289)
  line L160 (-9.0359, -50.0289) -> (-7.3038, -51.0289)
  line L161 (-5.5718, -50.0289) -> (-5.5718, -48.0289)
  line L162 (-7.1756, -45.2228) -> (-9.9918, -46.8487)
  line L163 (-8.8038, -44.4308) -> (-10.5359, -45.4308)
  line L164 (-10.5359, -45.4308) -> (-12.2679, -44.4308)
  line L165 (-8.8038, -43.4308) -> (-7.2869, -43.4308)
  line L166 (-8.8038, -42.4308) -> (-8.8038, -44.4308)
  line L167 (-12.2679, -44.4308) -> (-12.2679, -42.4308)
  line L168 (-12.2679, -42.4308) -> (-10.5359, -41.4308)
  line L169 (-10.5359, -41.4308) -> (-8.8038, -42.4308)
  line L170 (-7.1756, -41.6388) -> (-9.9918, -40.0129)
  line L171 (-9.0359, -59.225) -> (-7.3038, -58.225)
  line L172 (-9.0359, -60.225) -> (-9.8692, -60.225)
  line L173 (-9.0359, -61.225) -> (-9.0359, -59.225)
  line L174 (-7.3038, -62.225) -> (-9.0359, -61.225)
  line L175 (-5.5718, -61.225) -> (-7.3038, -62.225)
  line L176 (-5.5718, -59.225) -> (-5.5718, -61.225)
  line L177 (-7.3038, -58.225) -> (-5.5718, -59.225)
  line L178 (-7.1756, -56.4189) -> (-9.9918, -58.0448)
  line L179 (-10.5359, -67.8231) -> (-8.8038, -66.8231)
  line L180 (-12.2679, -66.8231) -> (-10.5359, -67.8231)
  line L181 (-8.8038, -65.8231) -> (-7.2869, -65.8231)
  line L182 (-8.8038, -66.8231) -> (-8.8038, -64.8231)
  line L183 (-12.2679, -64.8231) -> (-12.2679, -66.8231)
  line L184 (-8.8038, -64.8231) -> (-10.5359, -63.8231)
  line L185 (-10.5359, -63.8231) -> (-12.2679, -64.8231)
  line L186 (-10.5359, -90.2154) -> (-8.8038, -89.2154)
  line L187 (-12.2679, -89.2154) -> (-10.5359, -90.2154)
  line L188 (-8.8038, -88.2154) -> (-7.2869, -88.2154)
  line L189 (-12.2679, -87.2154) -> (-12.2679, -89.2154)
  line L190 (-8.8038, -89.2154) -> (-8.8038, -87.2154)
  line L191 (-10.5359, -86.2154) -> (-12.2679, -87.2154)
  line L192 (-8.8038, -87.2154) -> (-10.5359, -86.2154)
  line L193 (-10.5359, -75.0192) -> (-8.8038, -76.0192)
  line L194 (-8.8038, -78.0192) -> (-10.5359, -79.0192)
  line L195 (-8.8038, -77.0192) -> (-7.2869, -77.0192)
  line L196 (-10.5359, -79.0192) -> (-12.2679, -78.0192)
  line L197 (-8.8038, -76.0192) -> (-8.8038, -78.0192)
  line L198 (-12.2679, -76.0192) -> (-10.5359, -75.0192)
  line L199 (-12.2679, -78.0192) -> (-12.2679, -76.0192)
  line L200 (-10.5359, -101.4115) -> (-8.8038, -100.4115)
  line L201 (-12.2679, -100.4115) -> (-10.5359, -101.4115)
  line L202 (-8.8038, -99.4115) -> (-7.2869, -99.4115)
  line L203 (-8.8038, -100.4115) -> (-8.8038, -98.4115)
  line L204 (-8.8038, -98.4115) -> (-10.5359, -97.4115)
  line L205 (-10.5359, -97.4115) -> (-12.2679, -98.4115)
  line L206 (-12.2679, -98.4115) -> (-12.2679, -100.4115)
  line L207 (-10.5359, -123.8038) -> (-8.8038, -122.8038)
  line L208 (-12.2679, -122.8038) -> (-10.5359, -123.8038)
  line L209 (-8.8038, -121.8038) -> (-7.2869, -121.8038)
  line L210 (-8.8038, -122.8038) -> (-8.8038, -120.8038)
  line L211 (-8.8038, -120.8038) -> (-10.5359, -119.8038)
  line L212 (-10.5359, -119.8038) -> (-12.2679, -120.8038)
  line L213 (-12.2679, -120.8038) -> (-12.2679, -122.8038)
  point P0 (0, 0)
  point P1 (-26.6962, -15.4404)
  point P2 (-24.9641, -15.4404)
  dimension "d174" = 2
  dimension "d175" = 180
  dimension "d176" = 3
  dimension "d177" = 0
  dimension "d178" = 1.5
  dimension "d179" = 1.7321
  constraints: 422 end point, 238 symmetric about line, 4 midpoint, 3 horizontal, 1 parallel, 1 vertical, 13 other
  measures "d174" distance of L2.end L3.end
  measures "d175" angle of L6 L3
  measures "d176" distance from line of L7 point (-24.964, -15.44)
  measures "d177" vertical distance of L7.start L0.end
  measures "d178" distance between parallel lines of L1 L8
  measures "d179" distance between parallel lines of L101 L100
extrude "Extrusion59" cut sketch "Sketch8" against normal blind 2
sketch "Sketch9" plane through (0, 16.5, 0) normal (0, 1, 0) x (1, 0, 0)
  line L0 (-28.5684, -145) -> (-6.4316, -145) projected
  line L1 (-19.4999, -145) -> (-19.4999, -143)
  line L2 (-13, -143) -> (-22, -143) projected
  line L3 (-15.4999, -145) -> (-15.4999, -143)
  line L4 (-4.0696, 0) -> (-30.9304, 0) projected
  line L5 (-19.5002, 0) -> (-19.5002, -2)
  line L6 (-28.8957, -2) -> (-6.1043, -2) projected
  line L7 (-15.5002, 0) -> (-15.5002, -2)
  line L8 (-34.9298, -4.069) -> (-32.5678, -141.069) projected
  line L9 (-31.0773, -111.5) -> (-32.8951, -6.069) projected
  line L10 (-33.3187, -97.5178) -> (-31.319, -97.4834)
  line L11 (-33.2497, -101.5172) -> (-31.25, -101.4828)
  line L12 (-27.7, -111.5) -> (-31.0773, -111.5) projected
  line L13 (-34.9298, -4.069) -> (-32.5678, -141.069) projected
  line L14 (-34.0082, -57.5238) -> (-32.0085, -57.4893)
  line L15 (-34.0772, -53.5244) -> (-32.0775, -53.4899)
  line L16 (-2.1049, -6.069) -> (-3.9227, -111.5) projected
  line L17 (-2.4322, -141.069) -> (-0.0702, -4.069) projected
  line L18 (-3.681, -97.4834) -> (-1.6813, -97.5178)
  line L19 (-3.75, -101.4828) -> (-1.7503, -101.5172)
  line L20 (-3.9227, -111.5) -> (-7.3, -111.5) projected
  line L21 (-2.9915, -57.4893) -> (-0.9918, -57.5238)
  line L22 (-2.9225, -53.4899) -> (-0.9228, -53.5244)
  point P0 (0, 0)
  point P1 (-32.2499, -101.5)
  point P2 (-2.7501, -101.5)
  dimension "d182" = 4
  dimension "d183" = 9.0685
  dimension "d187" = 4
  dimension "d188" = 9.3955
  dimension "d189" = 4
  dimension "d190" = 10
  dimension "d191" = 4
  dimension "d192" = 40
  dimension "d193" = 4
  dimension "d194" = 10
  dimension "d195" = 4
  dimension "d196" = 40
  constraints: 24 end point, 22 point on line, 8 perpendicular, 4 vertical, 2 midpoint
  measures "d182" distance between parallel lines of L3 L1
  measures "d183" distance from line of L0.start L1
  measures "d187" distance between parallel lines of L7 L5
  measures "d188" distance from line of L6.start L5
  measures "d189" distance between parallel lines of L10 L11
  measures "d190" distance from line of L12 point (-32.25, -101.5)
  measures "d191" distance between parallel lines of L14 L15
  measures "d192" distance between parallel lines of L10 L14
  measures "d193" distance between parallel lines of L18 L19
  measures "d194" distance from line of L20 point (-2.75, -101.5)
  measures "d195" distance between parallel lines of L21 L22
  measures "d196" distance between parallel lines of L18 L21
extrude "Extrusion60" add sketch "Sketch9" along normal blind 3 contours L1 L2 L3 L0 | L7 L6 L5 L4 | L15 L9 L14 L8 | L10 L9 L11 L8 | L22 L17 L21 L16 | L18 L17 L19 L16
body "Solid1"
